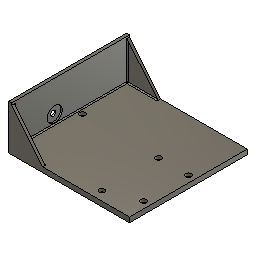
Radar RealSense Mount (Autodesk Fusion 360 design; units mm, degrees)
Autodesk Fusion 360 part; units mm, degrees
sketch "Sketch1" plane through (0, 0, 0) normal (0, 1, 0) x (1, 0, 0)
  line L0 (-50, 60) -> (70, 60)
  line L1 (70, 60) -> (70, -60)
  line L2 (70, -60) -> (-50, -60)
  line L3 (-50, -60) -> (-50, 60)
  dimension "d1" = 120
  constraint horizontal L0
  constraint vertical L1
  constraint horizontal L2
  constraint vertical L3
  measures "d1" distance of L0.start L0.end
extrude "Extrude1" add sketch "Sketch1" along normal blind 5
sketch "Sketch2" plane through (0, 5, 0) normal (0, 1, 0) x (-1, 0, 0)
  line L0 (50, 60) -> (-70, 60)
  line L1 (-70, 60) -> (-70, -60)
  line L2 (-70, -60) -> (50, -60)
  line L3 (50, -60) -> (50, 60)
  line L4 (50, -60) -> (47.5, -60)
  line L5 (47.5, -60) -> (47.5, 60)
  line L6 (47.5, 60) -> (50, 60)
  line L7 (50, 60) -> (50, -60)
  dimension "d4" = 2.5
  constraint horizontal L4
  constraint vertical L5
  constraint horizontal L6
  constraint vertical L7
  constraint coincident L2.end L3.start
  measures "d4" distance of L2.end L4.end
extrude "Extrude2" add sketch "Sketch2" along normal blind 40 contours L0 L2 L3 L4 L5 L6 L7
hole "Hole1" at (-47.5, 27.6902, 0.3168) direction (-1, 0, 0) diameter 6.35 depth 2.5 tip angle 180 counterbore diameter 14.7 counterbore depth 0.5
sketch "Sketch4" plane through (0, 5, 0) normal (0, 1, 0) x (-1, 0, 0)
  line L0 (47.5, -60) -> (47.5, 60)
  line L1 (47.5, 60) -> (-70, 60)
  line L2 (-70, 60) -> (-70, -60)
  line L3 (-70, -60) -> (47.5, -60)
  line L4 (47.5, 60) -> (44, 60)
  line L5 (41, 50) -> (47.5, 60)
  circle A0 centre (41, 50) radius 2.5
  line L6 (41, 50) -> (-35.3, 50)
  circle A1 centre (-35.3, 50) radius 2.5
  line L7 (41, 50) -> (41, -6.9)
  circle A2 centre (41, -6.9) radius 2.5
  line L8 (41, -6.9) -> (-35.3, -6.9)
  circle A3 centre (-35.3, -6.9) radius 2.5
  line L9 (-35.3, -6.9) -> (-65.3, -6.9)
  circle A4 centre (-65.3, -6.9) radius 2.5
  line L10 (-65.3, -6.9) -> (-65.3, 38.1)
  circle A5 centre (-65.3, 38.1) radius 2.5
  dimension "d15" = 5
  dimension "d16" = 76.3
  dimension "d17" = 5
  dimension "d18" = 56.9
  dimension "d19" = 5
  dimension "d20" = 76.3
  dimension "d21" = 5
  dimension "d22" = 30
  dimension "d23" = 5
  dimension "d24" = 45
  dimension "d25" = 5
  constraint coincident L0.end L1.start
  constraint coincident L1 L4.end
  constraint perpendicular L0 L4
  constraint coincident L5.start A0.centre
  constraint horizontal L6
  constraint coincident L6.end A1.centre
  constraint perpendicular L6 L7
  constraint coincident L7.end A2.centre
  constraint perpendicular L7 L8
  constraint coincident L8.end A3.centre
  constraint parallel L8 L9
  constraint coincident L9.end A4.centre
  constraint perpendicular L9 L10
  constraint coincident L10.end A5.centre
  measures "d15" diameter of A0
  measures "d16" distance of L5.start L6.end
  measures "d17" diameter of A1
  measures "d18" distance of L5.start L7.end
  measures "d19" diameter of A2
  measures "d20" distance of L7.end L8.end
  measures "d21" diameter of A3
  measures "d22" distance of L8.end L9.end
  measures "d23" diameter of A4
  measures "d24" distance of L9.end L10.end
  measures "d25" diameter of A5
hole "Hole2" at (-41, 5, -6.9) at (35.3, 5, -6.9) at (65.3, 5, -6.9) at (65.3, 5, 38.1) at (35.3, 5, 50) at (-41, 5, 50) direction (0, -1, 0) diameter 3 depth 5 tip angle 180 counterbore diameter 5 counterbore depth 3
sketch "Sketch5" plane through (0, 0, 60) normal (0, 0, 1) x (1, 0, 0)
  line L0 (-50, 0) -> (70, 0)
  line L1 (70, 0) -> (70, 5)
  line L2 (70, 5) -> (-47.5, 5)
  line L3 (-47.5, 5) -> (-47.5, 45)
  line L4 (-47.5, 45) -> (-50, 45)
  line L5 (-50, 45) -> (-50, 0)
  line L6 (-47.5, 45) -> (-15, 5)
  line L7 (-47.5, 5) -> (-47.5, 45)
  constraint coincident L3.end L4.start
  constraint coincident L2 L6.end
  constraint coincident L2.end L3.start
extrude "Extrude4" add sketch "Sketch5" against normal blind 2 contours L2 L3 L6 L7
sketch "Sketch6" plane through (0, 0, -60) normal (0, 0, -1) x (-1, 0, 0)
  line L0 (-70, 0) -> (50, 0)
  line L1 (50, 0) -> (50, 45)
  line L2 (50, 45) -> (47.5, 45)
  line L3 (47.5, 45) -> (47.5, 5)
  line L4 (47.5, 5) -> (-70, 5)
  line L5 (-70, 5) -> (-70, 0)
  line L6 (47.5, 45) -> (15, 5)
  line L7 (47.5, 5) -> (47.5, 45)
  constraint coincident L2.end L3.start
  constraint coincident L4 L6.end
  constraint coincident L3.end L4.start
extrude "Extrude5" add sketch "Sketch6" against normal blind 2 contours L3 L4 L6 L7
fillet "Fillet1" radius 1 7 edges at (-47.5, 5, 0) (-31.25, 5, 58) (-47.5, 25, 58) (-15, 5, 59) (-31.25, 5, -58) (-47.5, 25, -58) (-15, 5, -59)
extrude "Extrude6" cut 1 faces at (-50, 24.0723, -40.9409) along direction (1, 0, 0) blind 0.5
extrude "Extrude7" cut 1 faces at (-37.4334, 16.7898, 60) along direction (0, 0, -1) blind 0.5
extrude "Extrude8" cut 1 faces at (-37.4334, 16.7898, -60) along direction (0, 0, 1) blind 0.5
extrude "Extrude9" cut 1 faces at (70, 1.6667, -19.8333) along direction (-1, 0, 0) blind 0.5
extrude "Extrude10" cut 1 faces at (-37.4334, 16.7898, 59.5) along direction (0, 0, -1) blind 0.5
extrude "Extrude11" cut 1 faces at (-37.4334, 16.7898, -59.5) along direction (0, 0, 1) blind 0.5
extrude "Extrude12" cut 1 faces at (-49.5, 24.0723, -40.2743) along direction (1, 0, 0) blind 0.5
extrude "Extrude13" cut 1 faces at (69.5, 1.6667, -19.6667) along direction (-1, 0, 0) blind 0.5
delete_face "DeleteFace1" 9 faces at (-46.5747, 5.0028, -19) (-47.0459, 5.1724, -57.1305) (-25.3734, 5.0416, -57.2855) (-46.6258, 31.2753, -57.9921) (-14.8129, 5.0426, -57.8573) (-14.8129, 5.0426, 57.8573) (-25.3734, 5.0416, 57.2855) (-46.8897, 31.4869, 57.921) (-47.0459, 5.1724, 57.1305)
extrude "Extrude14" add 1 faces at (-36.6667, 18.3333, 58) along direction (0, 0, -1) blind 0.5
extrude "Extrude15" add 1 faces at (-47.5, 25.8967, -41.0111) along direction (1, 0, 0) blind 0.5
extrude "Extrude16" add 1 faces at (-36.3333, 18.1282, -58) along direction (0, 0, 1) blind 0.5
fillet "Fillet2" radius 1 5 edges at (-31, 5, -57.5) (-47, 5, 0) (-47, 24.6923, -57.5) (-31, 5, 57.5) (-47, 24.6923, 57.5)
sketch "Sketch7" plane through (-47, 0, 0) normal (1, 0, 0) x (0, 0, -1)
  line L0 (56.5, 44.3846) -> (58, 44.3846)
  line L1 (58, 44.3846) -> (58, 45)
  line L2 (58, 45) -> (-57.5, 45)
  line L3 (-57.5, 45) -> (-57.5, 44.3846)
  line L4 (-57.5, 44.3846) -> (-56.5, 44.3846)
  line L5 (-56.5, 44.3846) -> (-56.5, 6)
  line L6 (-56.5, 6) -> (56.5, 6)
  line L7 (56.5, 6) -> (56.5, 44.3846)
  circle A0 centre (-0.3168, 27.6902) radius 7.35
  line L8 (-0.3168, 27.6902) -> (-30, 27.6902)
  constraint coincident A0.centre L8.start
  constraint parallel L2 L8
hole "Hole3" at (-47, 27.6902, 30) direction (-1, 0, 0) diameter 5.118 depth 2 tip angle 180 counterbore diameter 15 counterbore depth 0.5
thread "Thread1" "ANSI Unified Screw Threads 0.25 1/4-20 UNC 1B"
extrude "Extrude17" add 1 faces at (-47.1667, 44.7949, -58) along direction (0, 0, -1) blind 1
extrude "Extrude18" add 1 faces at (-47.1667, 44.7949, 57.5) along direction (0, 0, 1) blind 1.5
delete_face "DeleteFace2" 2 faces at (-47.3333, 28.0566, -7.0241) (-48.6667, 28.0064, -2.8424)
move_face "MoveFace1" to x (1, 0, 0) y (0, 0.965926, -0.258819) z (0, 0.258819, 0.965926) at (0, -20.8163, 8.5548) 2 faces at (-48.1667, 25.8375, 31.7652) (-47.1667, 28.0641, 22.5093)
delete_face "DeleteFace3" 7 faces at (-46.0747, 5.0028, 18.8333) (-25.6586, 5.5942, 57.4139) (-46.5459, 5.1724, 56.6305) (-46.3897, 31.0766, 57.421) (-25.6586, 5.5942, -57.4139) (-46.1305, 5.1724, -57.0459) (-46.3897, 31.0766, -57.421)
extrude "Extrude19" add 1 faces at (-47, 21.4913, -30.6678) along direction (1, 0, 0) blind 1
extrude "Extrude20" add 1 faces at (-35.6667, 17.7179, 57.5) along direction (0, 0, -1) blind 1
extrude "Extrude21" add 1 faces at (-35.6667, 17.7179, -57.5) along direction (0, 0, 1) blind 1
extrude "Extrude22" add 1 faces at (-46.3333, 43.9744, 57.5) along direction (0, 0, 1) blind 1.5
extrude "Extrude23" add 1 faces at (-46.3333, 43.9744, -57.5) along direction (0, 0, -1) blind 1.5
delete_face "DeleteFace4" 12 faces at (35.813, 1.3333, -5.4905) (35.4246, 4, -4.4031) (66.155, 4, -9.2492) (64.7173, 1.3333, -5.5178) (64.7173, 1.3333, 39.4822) (66.155, 4, 35.7508) (35.813, 1.3333, 51.4095) (35.4246, 4, 52.4969) (-40.8754, 4, -4.4031) (-40.487, 1.3333, -5.4905) (-40.8754, 4, 52.4969) (-40.487, 1.3333, 51.4095)
hole "Hole4" at (35.3, 5, 50) at (65.3, 5, 38.1) at (65.3, 5, -6.9) at (35.3, 5, -6.9) at (-41, 5, -6.9) at (-41, 5, 50) direction (0, -1, 0) diameter 2.529 depth 5 tip angle 180 counterbore diameter 5.5 counterbore depth 3
thread "Thread2" "ANSI Metric M Profile 3.0 M3x0.5 6H"
fillet "Fillet3" radius 1 5 edges at (-30.5, 5, 56.5) (-46, 24.0769, 56.5) (-46, 5, 0) (-46, 24.0769, -56.5) (-30.5, 5, -56.5)
move_face "MoveFace2" to x (1, 0, 0) y (0, 0.939693, -0.34202) z (0, 0.34202, 0.939693) at (0, -9.7125, 2.5182) 2 faces at (-48, 13.1567, 27.8641) (-46.5, 12.1174, 23.0336)
move_face "MoveFace3" to x (1, 0, 0) y (0, 0.996195, -0.087156) z (0, 0.087156, 0.996195) at (0, -2.0525, -9.2089) 2 faces at (-48.5, 11.8731, 24.4291) (-46.5, 9.552, 20.0183)
extrude "Extrude24" add 1 faces at (69, 2.3333, -55.9362) along direction (1, 0, 0) blind 3
